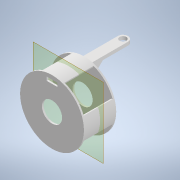
# Autodesk Inventor part: outer_part
Saved by Autodesk Inventor 2021 (Build 250183000, 183)
## iProperties
Created: 2022-07-01
Part Number: outer_part
Material: Типовые
Document SubType Name: Modeling
Designer: termi
Density: 1 g/cm^3
Appearance: По умолчанию
Author: termi
Autodesk Inventor part; units mm, degrees
ref_plane "YZ Plane" through (0, 0, 0) normal (1, 0, 0) x (0, 1, 0)
ref_plane "XZ Plane" through (0, 0, 0) normal (0, 1, 0) x (-1, 0, 0)
ref_plane "XY Plane" through (0, 0, 0) normal (0, 0, 1) x (1, 0, 0)
sketch "Эскиз1" plane through (0, 0, 0) normal (0, 1, 0) x (-1, 0, 0)
  line L0 (30, 181.2) -> (30, 186.2)
  line L1 (30, 186.2) -> (95, 186.2)
  line L2 (95, 186.2) -> (95, 90.2)
  line L3 (95, 90.2) -> (30, 90.2)
  line L4 (30, 90.2) -> (30, 95.2)
  line L5 (30, 95.2) -> (90, 95.2)
  line L6 (90, 95.2) -> (90, 181.2)
  line L7 (90, 181.2) -> (30, 181.2)
  line L8 (0, -115.5707) -> (0, 259.8393)
  line L9 (70, 181.2) -> (-70, 181.2) projected
  point P0 (0, 0)
  dimension "d0" = 5
  dimension "d1" = 5
  dimension "d2" = 5
  dimension "d3" = 86
  dimension "d4" = 180
  dimension "d5" = 60
  constraints: 18 end point, 5 perpendicular, 4 point on line, 2 vertical, 1 parallel
  measures "d0" distance between parallel lines of L7 L1
  measures "d1" distance between parallel lines of L3 L5
  measures "d2" distance between parallel lines of L2 L6
  measures "d3" distance between parallel lines of L5 L7
  measures "d4" diameter of L6 L8
  measures "d5" diameter of L3.end L8
revolve "Вращение1" add sketch "Эскиз1" angle 360 about axis through (0, 0, -115.5707) along (0, 0, 1)
sketch "Эскиз2" plane through (0, 0, 186.2) normal (0, 0, 1) x (1, 0, 0)
  line L0 (-15, 72.7645) -> (-15, 82.7645) projected
  line L1 (15, 82.7645) -> (-15, 82.7645) projected
  line L2 (15, 72.7645) -> (15, 82.7645) projected
  line L3 (-15, 72.7645) -> (15, 72.7645) projected
  line L4 (-15.5, 83.2645) -> (-15.5, 72.2645)
  line L5 (-15.5, 72.2645) -> (15.5, 72.2645)
  line L6 (15.5, 72.2645) -> (15.5, 83.2645)
  line L7 (15.5, 83.2645) -> (-15.5, 83.2645)
  point P0 (0, 0)
  dimension "d7" = 0.5
  constraints: 8 end point, 3 other
  measures "d7" distance between parallel lines of L1 L7
extrude "Выдавливание1" cut sketch "Эскиз2" against normal blind 7 contours L0 L1 L2 L3 | L7 L6 L5 L4
sketch "Эскиз3" plane through (0, 0, 90.2) normal (0, 0, -1) x (-1, 0, 0)
  line L0 (15, 82.7645) -> (-15, 82.7645) projected
  line L1 (-15, 72.7645) -> (15, 72.7645) projected
  line L2 (15, 72.7645) -> (15, 82.7645) projected
  line L3 (-15, 72.7645) -> (-15, 82.7645) projected
  point P0 (0, 0)
extrude "Выдавливание2" add sketch "Эскиз3" along normal blind 130
sketch "Эскиз4" plane through (-15, 82.7645, 90.2) normal (0, 1, 0) x (1, 0, 0)
  line L0 (30, 0) -> (30, 130) projected
  line L1 (0, 0) -> (0, 130) projected
  arc A0 (30, 115) -> (0, 115) centre (15, 115) ccw
  line L2 (30, 130) -> (0, 130) projected
  circle A1 centre (15, 115) radius 10
  point P0 (15, 90.2)
  point P1 (15, 130)
  dimension "d15" = 20
  constraints: 3 tangent, 2 centre point, 2 point on circle, 2 point on line, 1 coincident
  measures "d15" diameter of A1
extrude "Выдавливание3" cut sketch "Эскиз4" against normal blind 24.5
ref_plane "РабПлоскость1" through (0, 0, 138.2) normal (0, 0, -1) x (-1, 0, 0)
sketch "Эскиз5" plane through (0, 0, 138.2) normal (0, 0, -1) x (-1, 0, 0)
  line L0 (0, 0) -> (-41.3014, 113.4746)
  line L1 (-41.3014, 113.4746) -> (-113.4746, 41.3014)
  line L2 (-113.4746, 41.3014) -> (0, 0)
  line L3 (0, 0) -> (-77.388, 77.388) construction
  line L4 (0, 0) -> (-129.096, 0) construction
  dimension "d18" = 50
  dimension "d19" = 45
  constraints: 10 end point, 1 equal length, 1 horizontal, 1 midpoint
  measures "d18" angle of L0 L2
  measures "d19" angle of L3 L4
extrude "Выдавливание4" cut sketch "Эскиз5" along normal up to surface (43 mm away)
sketch "Эскиз6" plane through (0, 0, 138.2) normal (0, 0, -1) x (-1, 0, 0)
  arc A0 (-30.7818, 84.5723) -> (-84.5723, 30.7818) centre (0, 0) ccw projected
  line L0 (-30.7818, 84.5723) -> (-32.4919, 89.2708) projected
  arc A1 (-32.4919, 89.2708) -> (-89.2708, 32.4919) centre (0, 0) ccw projected
  line L1 (-89.2708, 32.4919) -> (-84.5723, 30.7818) projected
extrude "Выдавливание5" cut sketch "Эскиз6" against normal up to surface (43 mm away)
pattern_circular "Круговой массив1" count 4 over 360 about axis through (0, 0, 138.2) along (0, 0, -1) of "Выдавливание4", "Выдавливание5"
